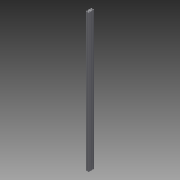
# Autodesk Inventor part: HammerStick Stick
Saved by Autodesk Inventor 2015 (Build 190159000, 159)
## iProperties
Created: 2015-01-13
Part Number: HammerStick Stick
Material: Generic
Document SubType Name: Modeling
Designer: harrykuperstein
Density: 1 g/cm^3
Appearance: Default
Mass: 1253.61 g
Surface Area: 3309.67 cm^2
Volume: 1253.61 cm^3
Author: harrykuperstein
Autodesk Inventor part; units mm, degrees
ref_plane "YZ Plane" through (0, 0, 0) normal (1, 0, 0) x (0, 1, 0)
ref_plane "XZ Plane" through (0, 0, 0) normal (0, 1, 0) x (-1, 0, 0)
ref_plane "XY Plane" through (0, 0, 0) normal (0, 0, 1) x (1, 0, 0)
sketch "Sketch1" plane through (0, 0, 0) normal (0, 1, 0) x (-1, 0, 0)
  line L0 (0, 0) -> (25.4, 0)
  line L1 (25.4, 0) -> (25.4, 50.8)
  line L2 (25.4, 50.8) -> (0, 50.8)
  line L3 (0, 50.8) -> (0, 0)
  dimension "d0" = 50.8
  dimension "d1" = 25.4
  constraints: 8 end point, 2 parallel, 1 horizontal, 1 perpendicular
  measures "d0" distance of L2.end L0.start
  measures "d1" distance of L0.start L0.end
extrude "Extrusion1" add sketch "Sketch1" along normal blind 1295.4
sketch "Sketch2" plane through (0, 0, 50.8) normal (0, 0, 1) x (1, 0, 0)
  line L0 (-9.525, 0) -> (-15.875, 0)
  line L1 (-15.875, 0) -> (-15.875, 1295.4)
  line L2 (-25.4, 0) -> (-25.4, 1295.4) projected
  line L3 (0, 1295.4) -> (-25.4, 1295.4) projected
  line L4 (-9.525, 1295.4) -> (-9.525, 0)
  line L5 (0, 0) -> (0, 1295.4) projected
  line L6 (0, 0) -> (-25.4, 0) projected
  line L7 (-15.875, 1295.4) -> (-9.525, 1295.4)
  dimension "d4" = 9.525
  dimension "d5" = 6.35
  dimension "d6" = 9.525
  dimension "d9" = 9.525
  constraints: 8 end point, 1 collinear, 1 parallel, 1 point on line, 1 vertical
  measures "d4" distance of L5.start L0.start
  measures "d5" distance of L0.start L0.end
  measures "d6" distance between parallel lines of L2 L1
  measures "d9" distance between parallel lines of L5 L4
extrude "Extrusion2" cut sketch "Sketch2" against normal blind 8.4667 contours L0 L1 L3 L4
sketch "Sketch3" plane through (-25.4, 0, 0) normal (0, 0, -1) x (-1, 0, 0)
  line L0 (-15.875, 0) -> (-9.525, 0)
  line L1 (-9.525, 0) -> (-9.525, 1295.4)
  line L2 (-9.525, 1295.4) -> (-15.875, 1295.4)
  line L3 (-15.875, 1295.4) -> (-15.875, 0)
  point P0 (-25.4, 0)
  constraints: 8 end point, 2 parallel, 1 horizontal, 1 perpendicular
extrude "Extrusion3" cut sketch "Sketch3" against normal blind 8.4667
sketch "Sketch4" plane through (-25.4, 0, 0) normal (-1, 0, 0) x (0, 0, 1)
  line L0 (0, 1295.4) -> (50.8, 1295.4) projected
  line L1 (9.525, 0) -> (15.875, 0)
  line L2 (15.875, 0) -> (15.875, 1295.4)
  line L3 (15.875, 1295.4) -> (9.525, 1295.4)
  line L4 (9.525, 1295.4) -> (9.525, 0)
  line L5 (35.9833, 1295.4) -> (42.3333, 1295.4)
  line L6 (42.3333, 1295.4) -> (42.3333, 0)
  line L7 (42.3333, 0) -> (35.9833, 0)
  line L8 (35.9833, 0) -> (35.9833, 1295.4)
  line L9 (0, 0) -> (0, 1295.4) projected
  point P0 (50.8, 0)
  dimension "d14" = 9.525
  dimension "d16" = 6.35
  dimension "d17" = 6.35
  dimension "d18" = 9.525
  constraints: 16 end point, 4 parallel, 2 horizontal, 2 perpendicular, 2 point on line
  measures "d14" distance of L9.start L1.start
  measures "d16" distance between parallel lines of L2 L4
  measures "d17" distance between parallel lines of L6 L8
  measures "d18" distance between parallel lines of L9 L4
extrude "Extrusion4" cut sketch "Sketch4" against normal blind 8.4667
sketch "Sketch5" plane through (0, 0, 50.8) normal (1, 0, 0) x (0, 0, -1)
  line L0 (8.4667, 0) -> (14.8167, 0)
  line L1 (14.8167, 0) -> (14.8167, 1295.4)
  line L2 (14.8167, 1295.4) -> (8.4667, 1295.4)
  line L3 (8.4667, 1295.4) -> (8.4667, 0)
  line L4 (34.925, 1295.4) -> (41.275, 1295.4)
  line L5 (41.275, 1295.4) -> (41.275, 0)
  line L6 (41.275, 0) -> (34.925, 0)
  line L7 (34.925, 0) -> (34.925, 1295.4)
  point P0 (50.8, 0)
  constraints: 16 end point, 4 parallel, 2 horizontal, 2 perpendicular
extrude "Extrusion5" cut sketch "Sketch5" against normal blind 8.4667
body "Solid1"
